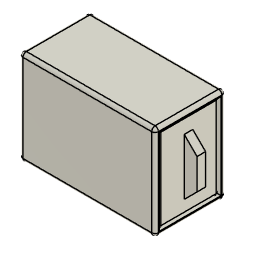
mtg-box-fusion (Autodesk Fusion 360 design; units mm, degrees)
Autodesk Fusion 360 part; units mm, degrees
note: some values were not read from the file. Set by a fixed rule: which sketch regions a step uses.
sketch "Sketch1" plane through (0, 0, 0) normal (0, 0, 1) x (1, 0, 0)
  line L0 (76, -35.5) -> (-76, -35.5)
  line L1 (-76, -35.5) -> (-76, 35.5)
  line L2 (-76, 35.5) -> (76, 35.5)
  line L3 (76, 35.5) -> (76, -35.5)
  line L4 (76, -35.5) -> (-76, 35.5) construction
  line L5 (-76, -35.5) -> (76, 35.5) construction
  line L6 (-73, 33.5) -> (-2.5, 33.5)
  line L7 (-2.5, 33.5) -> (-2.5, -33.5)
  line L8 (-2.5, -33.5) -> (-73, -33.5)
  line L9 (-73, -33.5) -> (-73, 33.5)
  line L10 (0.5, 33.5) -> (71, 33.5)
  line L11 (71, 33.5) -> (71, -33.5)
  line L12 (71, -33.5) -> (0.5, -33.5)
  line L13 (0.5, -33.5) -> (0.5, 33.5)
  dimension "d1" = 152
  dimension "d2" = 71
  dimension "d3" = 3
  dimension "d4" = 2
  dimension "d5" = 2
  dimension "d6" = 70.5
  dimension "d7" = 5
  dimension "d8" = 70.5
  constraint horizontal L0
  constraint perpendicular L0 L1
  constraint parallel L0 L2
  constraint parallel L1 L3
  constraint coincident L4 origin
  constraint coincident L5 origin
  constraint horizontal L6
  constraint vertical L7
  constraint horizontal L8
  constraint vertical L9
  constraint horizontal L10
  constraint vertical L11
  constraint horizontal L12
  constraint vertical L13
  constraint collinear L6 L10
  constraint collinear L8 L12
  measures "d1" distance of L1.end L2.end
  measures "d2" distance of L0.end L1.end
  measures "d3" distance of L1 L9
  measures "d4" distance of L2 L6
  measures "d5" distance of L0 L8
  measures "d6" distance of L7 L9
  measures "d7" distance of L3 L11
  measures "d8" distance of L11 L13
extrude "Extrude1" add sketch "Sketch1" along normal blind 98 makes body 1
extrude "Extrude2" add sketch "Sketch1" along normal blind 3 contours L6 L7 L8 L9 | L10 L11 L12 L13 bodies 1
sketch "Sketch2" plane through (0, 33.5, 0) normal (0, -1, 0) x (1, 0, 0)
  line L0 (-73, 3) -> (-2.5, 3)
  line L1 (-2.5, 3) -> (-2.5, 98)
  line L2 (-2.5, 98) -> (-73, 98)
  line L3 (-73, 98) -> (-73, 3)
  line L4 (-53, 98) -> (-22.5, 98)
  line L5 (-22.5, 98) -> (-22.5, 73)
  line L6 (-53, 73) -> (-53, 98)
  arc A0 (-53, 73) -> (-22.5, 73) centre (-37.75, 73) ccw
  dimension "d13" = 20
  dimension "d14" = 20
  dimension "d15" = 15.25
  dimension "d16" = 15.25
  dimension "d17" = 25
  constraint horizontal L4
  constraint vertical L5
  constraint vertical L6
  constraint coincident L2 L4.start
  measures "d13" distance of L3 L6
  measures "d14" distance of L1 L5
  measures "d15" distance of L6 A0.centre
  measures "d16" radius of A0
  measures "d17" distance of L2 A0.centre
extrude "Extrude3" cut sketch "Sketch2" along normal blind 90 and the other way blind 10 contours L2 L4 L5 L6 A0 bodies 1
sketch "Sketch3" plane through (0, 33.5, 0) normal (0, -1, 0) x (1, 0, 0)
  line L0 (0.5, 3) -> (71, 3)
  line L1 (71, 3) -> (71, 98)
  line L2 (71, 98) -> (0.5, 98)
  line L3 (0.5, 98) -> (0.5, 3)
  line L4 (20.5, 98) -> (51, 98)
  line L5 (51, 98) -> (51, 73)
  line L6 (20.5, 73) -> (20.5, 98)
  arc A0 (20.5, 73) -> (51, 73) centre (35.75, 73) ccw
  dimension "d22" = 20
  dimension "d23" = 20
  dimension "d24" = 25
  dimension "d25" = 15.25
  dimension "d31" = 25
  constraint horizontal L4
  constraint vertical L5
  constraint vertical L6
  constraint coincident L2 L4.start
  measures "d22" distance of L3 L6
  measures "d23" distance of L1 L5
  measures "d24" distance of L4.end L5.end
  measures "d25" radius of A0
  measures "d31" distance of L2 A0.centre
extrude "Extrude4" cut sketch "Sketch3" along normal blind 70 and the other way blind 5 contours L2 L4 L5 L6 A0 bodies 1
sketch "Sketch4" plane through (0, -35.5, 0) normal (0, -1, 0) x (1, 0, 0)
  line L0 (51, 98) -> (51, 73)
  arc A0 (20.5, 73) -> (51, 73) centre (35.75, 73) ccw
  line L1 (20.5, 73) -> (20.5, 98)
  line L2 (20.5, 98) -> (-22.5, 98)
  line L3 (-22.5, 98) -> (-22.5, 73)
  arc A1 (-53, 73) -> (-22.5, 73) centre (-37.75, 73) ccw
  line L4 (-53, 73) -> (-53, 98)
  line L5 (-53, 98) -> (-76, 98)
  line L6 (-76, 98) -> (-76, 0)
  line L7 (-76, 0) -> (76, 0)
  line L8 (76, 0) -> (76, 98)
  line L9 (76, 98) -> (51, 98)
  line L10 (76, 35) -> (20, 35)
  line L11 (20, 35) -> (20, 48)
  line L12 (20, 48) -> (76, 48)
  line L13 (21.5, 46.5) -> (51, 46.5)
  line L14 (51, 36.5) -> (21.5, 36.5)
  line L15 (21.5, 36.5) -> (21.5, 46.5)
  line L16 (51, 46.5) -> (51, 48)
  line L17 (51, 36.5) -> (51, 35)
  line L18 (31.5, 46.5) -> (31.5, 36.5)
  dimension "d32" = 50
  dimension "d33" = 35
  dimension "d34" = 56
  dimension "d35" = 25
  dimension "d36" = 1.5
  dimension "d37" = 1.5
  dimension "d38" = 1.5
  dimension "d39" = 25
  dimension "d40" = 25
  dimension "d41" = 10
  constraint parallel L10 L12
  constraint coincident L8 L10.start
  constraint coincident L8 L12.end
  constraint horizontal L13
  constraint horizontal L14
  constraint vertical L15
  constraint coincident L12 L16.end
  constraint perpendicular L12 L16
  constraint coincident L10 L17.end
  constraint perpendicular L10 L17
  constraint coincident L13 L18.start
  constraint coincident L14 L18.end
  constraint perpendicular L14 L18
  measures "d32" distance of L8.end L12.end
  measures "d33" distance of L7.end L10.start
  measures "d34" distance of L8 L11
  measures "d35" distance of A0.centre L12
  measures "d36" distance of L11 L15
  measures "d37" distance of L12 L13
  measures "d38" distance of L10 L14
  measures "d39" distance of L8 L16
  measures "d40" distance of L8 L17
  measures "d41" distance of L15 L18
extrude "Extrude5" cut sketch "Sketch4" against normal blind 75 contours L10 L11 L12 L13 L14 L15 L16 L17 bodies 1
sketch "Sketch5" plane through (0, 0, 36.5) normal (0, 0, -1) x (1, 0, 0)
  line L0 (21.5, 33.5) -> (51, 33.5)
  line L1 (51, 33.5) -> (51, 35.5)
  line L2 (51, 35.5) -> (21.5, 35.5)
  line L3 (21.5, 35.5) -> (21.5, 33.5)
  line L4 (21.5, 35.5) -> (24.5, 37.5)
  line L5 (24.5, 37.5) -> (27.5, 35.5)
  circle A0 centre (24.5, 34.25) radius 3.25
  dimension "d44" = 2
  dimension "d45" = 6
  constraint coincident L2.end L3.start
  constraint coincident L2 L5.end
  constraint equal L4 L5
  constraint coincident L2.end A0
  constraint coincident L4.end A0
  constraint coincident L5.end A0
  measures "d44" distance of L2 L4.end
  measures "d45" distance of L2.end L5.end
extrude "Extrude6" add sketch "Sketch5" against normal blind 10 contours L2 L4 L5 | L4 A0 | L5 A0 bodies 1
sketch "Sketch6" plane through (0, 0, 36.5) normal (0, 0, -1) x (1, 0, 0)
  line L0 (51, -35.5) -> (51, -33.5)
  line L1 (51, -33.5) -> (21.5, -33.5)
  line L2 (21.5, -33.5) -> (21.5, -35.5)
  line L3 (21.5, -35.5) -> (24.5, -37.5)
  line L4 (24.5, -37.5) -> (27.5, -35.5)
  circle A0 centre (24.5, -34.25) radius 3.25
  line L5 (21.5, -35.5) -> (51, -35.5)
  dimension "d48" = 6
  dimension "d52" = 2
  dimension "d53" = 6.5
  constraint coincident L2.end L3.start
  constraint equal L3 L4
  constraint coincident L4.end A0
  constraint coincident L3.end A0
  constraint coincident L2.end A0
  measures "d48" distance of L2.end L4.end
  measures "d52" distance of L3.end L5
  measures "d53" diameter of A0
extrude "Extrude7" add sketch "Sketch6" against normal blind 10 contours L4 A0 | L3 L4 L5 | L3 A0 bodies 1
sketch "Sketch7" plane through (76, 0, 0) normal (1, 0, 0) x (0, 1, 0)
  line L0 (-35.5, 0) -> (35.5, 0)
  line L1 (35.5, 0) -> (35.5, 98)
  line L2 (35.5, 98) -> (-35.5, 98)
  line L3 (-35.5, 98) -> (-35.5, 0)
  line L4 (-5, 82) -> (5, 82)
  line L5 (5, 82) -> (5, 16)
  line L6 (5, 16) -> (-5, 16)
  line L7 (-5, 16) -> (-5, 82)
  dimension "d54" = 10
  dimension "d55" = 16
  dimension "d56" = 16
  dimension "d57" = 30.5
  constraint horizontal L4
  constraint vertical L5
  constraint horizontal L6
  constraint vertical L7
  measures "d54" distance of L5 L7
  measures "d55" distance of L0 L6
  measures "d56" distance of L2 L4
  measures "d57" distance of L1 L5
extrude "Extrude8" add sketch "Sketch7" along normal blind 15 contours L4 L5 L6 L7 bodies 1
chamfer "Chamfer1" distance 15 angle 45 1 edges at (91, 0, 82) on bodies 1
chamfer "Chamfer2" distance 15 angle 45 1 edges at (91, 0, 16) on bodies 1
fillet "Fillet5" radius 1 1 edges at (21.5, -33.5, 41.5) on bodies 1
fillet "Fillet6" radius 1 1 edges at (21.5, 33.5, 41.5) on bodies 1
fillet "Fillet7" radius 3 8 edges at (0, -35.5, 0) (-76, 0, 0) (76, 0, 0) (0, 35.5, 0) (76, 35.5, 49) (76, -35.5, 49) (-76, 35.5, 49) (-76, -35.5, 49) on bodies 1
copy_body "Body->Comp1" bodies 1 removing the originals makes body 2 in component "tray"
ref_plane "WorkPlane1" through (-73, 0, 50.5) normal (-1, 0, 0) x (0, -1, 0)
sketch "Sketch8" plane through (-73, 0, 0) normal (-1, 0, 0) x (0, -1, 0)
  line L0 (36.25, 100) -> (-36.25, 100)
  line L1 (-36.25, 100) -> (-36.25, -0.75)
  line L2 (-36.25, -0.75) -> (36.25, -0.75)
  line L3 (36.25, -0.75) -> (36.25, 100)
  line L4 (33.5, 98) -> (-33.5, 98)
  line L5 (35.5, 3) -> (35.5, 98)
  line L6 (-33.5, 3) -> (-33.5, 98)
  line L7 (-32.5, 0) -> (32.5, 0)
  line L8 (-35.5, 98) -> (-35.5, 3)
  line L9 (41.25, 105) -> (-41.25, 105)
  line L10 (-41.25, 105) -> (-41.25, -5.75)
  line L11 (-41.25, -5.75) -> (41.25, -5.75)
  line L12 (41.25, -5.75) -> (41.25, 105)
  dimension "d77" = 2
  dimension "d78" = 0.75
  dimension "d80" = 0.75
  dimension "d81" = 0.75
  dimension "d82" = 5
  dimension "d83" = 5
  dimension "d84" = 5
  dimension "d85" = 5
  constraint horizontal L0
  constraint vertical L1
  constraint horizontal L2
  constraint vertical L3
  constraint horizontal L9
  constraint vertical L10
  constraint horizontal L11
  constraint vertical L12
  measures "d77" distance of L0 L4
  measures "d78" distance of L3 L5
  measures "d80" distance of L2 L7
  measures "d81" distance of L1 L8
  measures "d82" distance of L0 L9
  measures "d83" distance of L2 L11
  measures "d84" distance of L3 L12
  measures "d85" distance of L1 L10
extrude "Extrude9" add sketch "Sketch8" along normal blind 10 and the other way blind 149 separate body makes body 3
sketch "Sketch9" plane through (0, 0, 100) normal (0, 0, -1) x (1, 0, 0)
  line L0 (76, 36.25) -> (-83, 36.25)
  line L1 (-83, 36.25) -> (-83, -36.25)
  line L2 (-83, -36.25) -> (76, -36.25)
  line L3 (76, -36.25) -> (76, 36.25)
  line L4 (-83, 36.25) -> (-78, 36.25)
  line L5 (-78, 36.25) -> (-78, -36.25)
  line L6 (-78, -36.25) -> (-83, -36.25)
  line L7 (-83, -36.25) -> (-83, 36.25)
  dimension "d90" = 5
  constraint horizontal L4
  constraint vertical L5
  constraint horizontal L6
  constraint vertical L7
  constraint coincident L0.end L1.start
  measures "d90" distance of L0.end L4.end
extrude "Extrude10" add sketch "Sketch9" along normal blind 101 contours L0 L1 L2 L4 L5 L6 L7 bodies 3
ref_plane "WorkPlane2" through (0, -35.5, 50.5) normal (0, -1, 0) x (1, 0, 0)
sketch "Sketch10" plane through (0, -35.5, 0) normal (0, -1, 0) x (-1, 0, 0)
  line L0 (-21.5, -46.5) -> (-27.5, -46.5)
  line L1 (-27.5, -46.5) -> (-27.5, -36.5)
  line L2 (-27.5, -36.5) -> (-21.5, -36.5)
  line L3 (-21.5, -36.5) -> (-21.5, -46.5)
  line L4 (-20.75, -47.25) -> (-28.25, -47.25)
  line L5 (-28.25, -47.25) -> (-28.25, -35.75)
  line L6 (-28.25, -35.75) -> (-20.75, -35.75)
  line L7 (-20.75, -35.75) -> (-20.75, -47.25)
  line L8 (-76, -105) -> (-76, 5.75)
  line L9 (83, 5.75) -> (-76, 5.75)
  dimension "d94" = 48.5
  dimension "d95" = 42.25
  dimension "d96" = 6
  dimension "d97" = 10
  dimension "d98" = 0.75
  dimension "d99" = 0.75
  dimension "d100" = 0.75
  dimension "d101" = 0.75
  constraint horizontal L0
  constraint vertical L1
  constraint horizontal L2
  constraint vertical L3
  constraint horizontal L4
  constraint vertical L5
  constraint horizontal L6
  constraint vertical L7
  measures "d94" distance of L1 L8
  measures "d95" distance of L2 L9
  measures "d96" distance of L1 L3
  measures "d97" distance of L0 L2
  measures "d98" distance of L0 L4
  measures "d99" distance of L3 L7
  measures "d100" distance of L1 L5
  measures "d101" distance of L2 L6
extrude "Extrude11" cut sketch "Sketch10" along normal blind 2 from surface at 0.75 contours L0 L1 L2 L3 | L4 L5 L6 L7 bodies 3
ref_plane "WorkPlane3" through (0, 35.5, 50.5) normal (0, 1, 0) x (-1, 0, 0)
sketch "Sketch11" plane through (0, 35.5, 0) normal (0, 1, 0) x (1, 0, 0)
  line L0 (27.5, -46.5) -> (21.5, -46.5)
  line L1 (21.5, -46.5) -> (21.5, -36.5)
  line L2 (21.5, -36.5) -> (27.5, -36.5)
  line L3 (27.5, -36.5) -> (27.5, -46.5)
  line L4 (28.25, -47.25) -> (20.75, -47.25)
  line L5 (20.75, -47.25) -> (20.75, -35.75)
  line L6 (20.75, -35.75) -> (28.25, -35.75)
  line L7 (28.25, -35.75) -> (28.25, -47.25)
  line L8 (76, 5.75) -> (76, -105)
  line L9 (76, 5.75) -> (-83, 5.75)
  dimension "d106" = 48.5
  dimension "d107" = 42.25
  dimension "d108" = 6
  dimension "d109" = 10
  dimension "d110" = 0.75
  dimension "d111" = 0.75
  dimension "d112" = 0.75
  dimension "d113" = 0.75
  constraint horizontal L0
  constraint vertical L1
  constraint horizontal L2
  constraint vertical L3
  constraint horizontal L4
  constraint vertical L5
  constraint horizontal L6
  constraint vertical L7
  measures "d106" distance of L3 L8
  measures "d107" distance of L2 L9
  measures "d108" distance of L1 L3
  measures "d109" distance of L0 L2
  measures "d110" distance of L0 L4
  measures "d111" distance of L3 L7
  measures "d112" distance of L2 L6
  measures "d113" distance of L1 L5
extrude "Extrude12" cut sketch "Sketch11" along normal blind 2 from surface at 0.75 contours L0 L1 L2 L3 | L4 L5 L6 L7 bodies 3
copy_body "Body->Comp2" bodies 3 removing the originals makes body 4 in component "cover"
fillet "Fillet1" radius 4 12 edges at (76, 41.25, 49.625) (76, -41.25, 49.625) (-83, 41.25, 49.625) (-83, -41.25, 49.625) (-3.5, -41.25, -5.75) (-3.5, 41.25, -5.75) (-3.5, 41.25, 105) (-3.5, -41.25, 105) (76, 0, 105) (76, 0, -5.75) (-83, 0, 105) (-83, 0, -5.75) on bodies 4 in component "cover"
sketch "Sketch12" plane through (0, 0, 0) normal (0, 0, 1) x (1, 0, 0)
  line L0 (34.5, -46.75) -> (-34.5, -46.75)
  line L1 (-34.5, -46.75) -> (-34.5, 46.75)
  line L2 (-34.5, 46.75) -> (34.5, 46.75)
  line L3 (34.5, 46.75) -> (34.5, -46.75)
  line L4 (34.5, -46.75) -> (-34.5, 46.75) construction
  line L5 (-34.5, -46.75) -> (34.5, 46.75) construction
  line L6 (-31.5, 43.75) -> (31.5, 43.75)
  line L7 (31.5, 43.75) -> (31.5, -43.75)
  line L8 (31.5, -43.75) -> (-31.5, -43.75)
  line L9 (-31.5, -43.75) -> (-31.5, 43.75)
  line L10 (-32.5, 44.75) -> (32.5, 44.75)
  line L11 (32.5, 44.75) -> (32.5, -44.75)
  line L12 (32.5, -44.75) -> (-32.5, -44.75)
  line L13 (-32.5, -44.75) -> (-32.5, 44.75)
  dimension "d125" = 69
  dimension "d126" = 93.5
  dimension "d134" = 3
  dimension "d135" = 3
  dimension "d136" = 3
  dimension "d137" = 3
  dimension "d138" = 1
  dimension "d139" = 1
  dimension "d140" = 1
  dimension "d141" = 1
  constraint horizontal L0
  constraint perpendicular L0 L1
  constraint parallel L0 L2
  constraint parallel L1 L3
  constraint coincident L4 origin
  constraint coincident L5 origin
  constraint horizontal L6
  constraint vertical L7
  constraint horizontal L8
  constraint vertical L9
  constraint horizontal L10
  constraint vertical L11
  constraint horizontal L12
  constraint vertical L13
  measures "d125" distance of L1.end L2.end
  measures "d126" distance of L0.end L1.end
  measures "d134" distance of L3 L7
  measures "d135" distance of L0 L8
  measures "d136" distance of L1 L9
  measures "d137" distance of L2 L6
  measures "d138" distance of L8 L12
  measures "d139" distance of L9 L13
  measures "d140" distance of L6 L10
  measures "d141" distance of L7 L11
extrude "Extrude13" add sketch "Sketch12" along normal blind 20 separate body contours L10 L11 L12 L13 makes body 5
extrude "Extrude14" add sketch "Sketch12" along normal blind 3 contours L6 L7 L8 L9 bodies 5
extrude "Extrude15" add sketch "Sketch12" along normal blind 12 contours L0 L1 L2 L3 bodies 5
copy_body "CopyPasteBodies1" bodies 5 makes body 6
move_body "Move1" bodies 6 to x (1, 0, 0) y (0, 1, 0) z (0, 0, 1) at (-80, 0, 0)
extrude "Extrude16" cut 1 faces at (-112.1667, 14.5833, 20) along direction (0, 0, -1) blind 10 on bodies 6 bodies 6
extrude "Extrude17" add 1 faces at (-113.8333, 14.9167, 12) along direction (0, 0, 1) blind 10 on bodies 6 bodies 6
extrude "Extrude18" cut 1 faces at (-113.8333, 14.9167, 22) along direction (0, 0, -1) blind 4 on bodies 6 bodies 6
extrude "Extrude19" cut 1 faces at (-112.1667, 14.5833, 10) along direction (0, 0, -1) blind 0.5 on bodies 6 bodies 6
fillet "Fillet8" radius 2 16 edges at (0, -46.75, 0) (-34.5, 0, 0) (34.5, 0, 0) (0, 46.75, 0) (34.5, -46.75, 6) (-34.5, -46.75, 6) (34.5, 46.75, 6) (-34.5, 46.75, 6) (-80, -46.75, 0) (-45.5, 0, 0) (-114.5, 0, 0) (-80, 46.75, 0) (-114.5, -46.75, 9) (-45.5, -46.75, 9) (-45.5, 46.75, 9) (-114.5, 46.75, 9) on bodies 5 6
extrude "Extrude20" cut 1 faces at (-112.5, -14.9167, 12.3333) along direction (-1, 0, 0) blind 0.3 on bodies 6 bodies 6
extrude "Extrude21" cut 1 faces at (-91.0333, 44.75, 12.3333) along direction (0, 1, 0) blind 0.3 on bodies 6 bodies 6
extrude "Extrude22" cut 1 faces at (-47.5, 15.1167, 15.1667) along direction (1, 0, 0) blind 0.3 on bodies 6 bodies 6
extrude "Extrude23" cut 1 faces at (-69.0667, -44.75, 12.3333) along direction (0, -1, 0) blind 0.3 on bodies 6 bodies 6
copy_body "Body->Comp3" bodies 5 removing the originals makes body 7 in component "dice_tray"
copy_body "Body->Comp4" bodies 6 removing the originals makes body 8 in component "dice_cover"
component "tray" placed x (1, 0, 0) y (0, 1, 0) z (0, 0, 1) at (0, 0, 0)
component "cover" placed x (1, 0, 0) y (0, 1, 0) z (0, 0, 1) at (2, 0, 0.875)
component "dice_tray" placed x (1, 0, 0) y (0, 0, 1) z (0, -1, 0) at (-37.75, 33.5, 50.5)
component "dice_cover" placed x (1, 0, 0) y (0, 0, -1) z (0, 1, 0) at (42.25, 3.5, 50.5)
named bodies: "tray", "cover", "dice_tray", "dice_cover"
